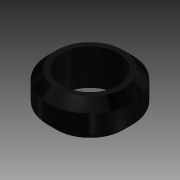
# Autodesk Inventor part: Solid V-Wheel
Saved by Autodesk Inventor 2014 SP1 (Build 180222100, 222)
## iProperties
Created: 2016-04-09
Part Number: Solid V-Wheel
Material: Generic
Document SubType Name: Modeling
Designer: Ben
Density: 1 g/cm^3
Appearance: Default
Author: Ben
Autodesk Inventor part; units mm, degrees
ref_plane "YZ Plane" through (0, 0, 0) normal (1, 0, 0) x (0, 1, 0)
ref_plane "XZ Plane" through (0, 0, 0) normal (0, 1, 0) x (-1, 0, 0)
ref_plane "XY Plane" through (0, 0, 0) normal (0, 0, 1) x (1, 0, 0)
sketch "Sketch1" plane through (0, 0, 0) normal (0, 0, 1) x (1, 0, 0)
  line L0 (0, 0) -> (0, 12.4297) construction
  line L1 (7.987, 0) -> (9.487, 0)
  line L2 (9.487, 0) -> (11.95, 2.463)
  line L3 (11.95, 7.767) -> (9.487, 10.23)
  line L4 (9.487, 10.23) -> (7.987, 10.23)
  line L5 (7.987, 10.23) -> (7.987, 0)
  line L6 (7.987, 5.115) -> (38.026, 5.115) construction
  line L7 (0, 0) -> (31.3179, 0) construction
  line L8 (11.95, 7.767) -> (11.95, 2.463)
  point P0 (8.9576, 5.115)
  dimension "d0" = 10.23
  dimension "d1" = 15.974
  dimension "d2" = 90
  dimension "d5" = 23.9
  dimension "d7" = 1.5
  constraints: 18 end point, 5 perpendicular, 1 collinear, 1 midpoint, 1 parallel, 1 point on line, 1 vertical, 1 other
  measures "d0" distance of L4.end L1.start
  measures "d1" diameter of L5 L0
  measures "d2" angle of L2 L3
  measures "d5" diameter of L3.start L0
  measures "d7" distance of L1.start L1.end
revolve "Revolution1" add sketch "Sketch1" angle 360 about axis through (0, 0, 0) along (0, 1, 0)
body "Solid1"
